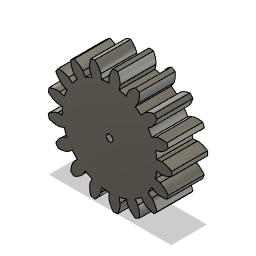
Gear v1 (Autodesk Fusion 360 design; units mm, degrees)
Autodesk Fusion 360 part; units mm, degrees
note: some values were not read from the file. Set by a fixed rule: which sketch regions a step uses.
(part 1 of 6)
sketch "Sketch1" plane through (0, 0, 0) normal (0, 0, 1) x (1, 0, 0)
  spline S0 degree 5 poles (16.3808, -1.6095) (16.3809, -1.6096) (16.3812, -1.6096) (16.3817, -1.6096) (16.3824, -1.6097) (16.3835, -1.6098) (16.3848, -1.6099) (16.3862, -1.61) (16.3879, -1.6101) (16.3897, -1.6102) (16.3916, -1.6103) (16.3937, -1.6104) (16.396, -1.6106) (16.3984, -1.6107) (16.401, -1.6108) (16.4037, -1.6109) (16.4066, -1.6111) (16.4096, -1.6112) (16.4128, -1.6113) (16.4161, -1.6114) (16.4195, -1.6115) (16.4231, -1.6116) (16.4268, -1.6117) (16.4306, -1.6118) (16.4346, -1.6118) (16.4387, -1.6119) (16.443, -1.6119) (16.4473, -1.612) (16.4518, -1.612) (16.4564, -1.612) (16.4611, -1.612) (16.466, -1.612) (16.471, -1.612) (16.476, -1.6119) (16.4812, -1.6119) (16.4866, -1.6118) (16.492, -1.6117) (16.4975, -1.6116) (16.5032, -1.6115) (16.5089, -1.6113) (16.5148, -1.6111) (16.5207, -1.6109) (16.5268, -1.6107) (16.533, -1.6105) (16.5393, -1.6103) (16.5456, -1.61) (16.5521, -1.6097) (16.5587, -1.6094) (16.5654, -1.609) (16.5722, -1.6087) (16.579, -1.6083) (16.586, -1.6079) (16.5931, -1.6074) (16.6002, -1.607) (16.6075, -1.6065) (16.6148, -1.606) (16.6222, -1.6054) (16.6298, -1.6049) (16.6374, -1.6043) (16.6451, -1.6036) (16.6528, -1.603) (16.6607, -1.6023) (16.6687, -1.6016) (16.6767, -1.6009) (16.6848, -1.6001) (16.693, -1.5993) (16.7013, -1.5985) (16.7097, -1.5977) (16.7181, -1.5968) (16.7267, -1.5959) (16.7353, -1.5949) (16.744, -1.594) (16.7527, -1.593) (16.7616, -1.5919) (16.7705, -1.5909) (16.7795, -1.5898) (16.7885, -1.5886) (16.7977, -1.5875) (16.8069, -1.5863) (16.8162, -1.585) (16.8256, -1.5838) (16.835, -1.5825) (16.8445, -1.5812) (16.8541, -1.5798) (16.8637, -1.5784) (16.8734, -1.577) (16.8832, -1.5755) (16.8931, -1.574) (16.903, -1.5725) (16.913, -1.5709) (16.923, -1.5693) (16.9331, -1.5676) (16.9433, -1.566) (16.9536, -1.5643) (16.9639, -1.5625) (16.9742, -1.5607) (16.9847, -1.5589) (16.9952, -1.557) (17.0057, -1.5552) (17.0164, -1.5532) (17.0271, -1.5512) (17.0378, -1.5492) (17.0486, -1.5472) (17.0595, -1.5451) (17.0704, -1.543) (17.0814, -1.5408) (17.0924, -1.5386) (17.1035, -1.5364) (17.1147, -1.5341) (17.1259, -1.5318) (17.1372, -1.5295) (17.1485, -1.5271) (17.1599, -1.5247) (17.1713, -1.5222) (17.1828, -1.5197) (17.1944, -1.5171) (17.206, -1.5146) (17.2176, -1.5119) (17.2293, -1.5093) (17.2411, -1.5066) (17.2529, -1.5038) (17.2647, -1.501) (17.2767, -1.4982) (17.2886, -1.4953) (17.3006, -1.4924) (17.3127, -1.4895) (17.3248, -1.4865) (17.337, -1.4835) (17.3492, -1.4804) (17.3614, -1.4773) (17.3738, -1.4741) (17.3861, -1.4709) (17.3985, -1.4677) (17.411, -1.4644) (17.4235, -1.4611) (17.436, -1.4578) (17.4486, -1.4544) (17.4612, -1.4509) (17.4739, -1.4474) (17.4866, -1.4439) (17.4994, -1.4403) (17.5122, -1.4367) (17.5251, -1.4331) (17.538, -1.4294) (17.5509, -1.4256) (17.5639, -1.4218) (17.5769, -1.418) (17.59, -1.4141) (17.6031, -1.4102) (17.6163, -1.4063) (17.6295, -1.4023) (17.6427, -1.3982) (17.656, -1.3942) (17.6693, -1.39) (17.6827, -1.3859) (17.696, -1.3816) (17.7095, -1.3774) (17.723, -1.3731) (17.7365, -1.3687) (17.75, -1.3643) (17.7636, -1.3599) (17.7772, -1.3554) (17.7909, -1.3509) (17.8046, -1.3463) (17.8183, -1.3417) (17.8321, -1.3371) (17.8459, -1.3324) (17.8598, -1.3276) (17.8736, -1.3229) (17.8876, -1.318) (17.9015, -1.3131) (17.9155, -1.3082) (17.9295, -1.3033) (17.9436, -1.2982) (17.9577, -1.2932) (17.9718, -1.2881) (17.9859, -1.283) (18.0001, -1.2778) (18.0143, -1.2725) (18.0286, -1.2672) (18.0429, -1.2619) (18.0572, -1.2566) (18.0716, -1.2511) (18.0859, -1.2457) (18.1004, -1.2402) (18.1148, -1.2346) (18.1293, -1.229) (18.1438, -1.2234) (18.1583, -1.2177) (18.1729, -1.212) (18.1875, -1.2062) (18.2021, -1.2004) (18.2167, -1.1945) (18.2314, -1.1886) (18.2461, -1.1826) (18.2609, -1.1766) (18.2756, -1.1706) (18.2904, -1.1645) (18.3053, -1.1583) (18.3201, -1.1521) (18.335, -1.1459) (18.3499, -1.1396) (18.3648, -1.1333) (18.3798, -1.1269) (18.3948, -1.1205) (18.4098, -1.114) (18.4248, -1.1075) (18.4399, -1.101) (18.4549, -1.0943) (18.4701, -1.0877) (18.4852, -1.081) (18.5004, -1.0743) (18.5155, -1.0675) (18.5307, -1.0606) (18.546, -1.0537) (18.5612, -1.0468) (18.5765, -1.0398) (18.5918, -1.0328) (18.6071, -1.0257) (18.6225, -1.0186) (18.6379, -1.0115) (18.6533, -1.0043) (18.6687, -0.997) (18.6841, -0.9897) (18.6996, -0.9824) (18.7151, -0.975) (18.7306, -0.9675) (18.7461, -0.96) (18.7616, -0.9525) (18.7772, -0.9449) (18.7928, -0.9373) (18.8084, -0.9296) (18.824, -0.9219) (18.8397, -0.9141) (18.8553, -0.9063) (18.871, -0.8984) (18.8867, -0.8905) (18.9024, -0.8826) (18.9182, -0.8746) (18.9339, -0.8665) (18.9497, -0.8584) (18.9624, -0.8519) (18.9718, -0.847) (18.9782, -0.8437) (18.9813, -0.8421) knots 0 0 0 0 0 0 0.00416667 0.00833333 0.0125 0.01666667 0.02083333 0.025 0.02916667 0.03333333 0.0375 0.04166667 0.04583333 0.05 0.05416667 0.05833333 0.0625 0.06666667 0.07083333 0.075 0.07916667 0.08333333 0.0875 0.09166667 0.09583333 0.1 0.10416667 0.10833333 0.1125 0.11666667 0.12083333 0.125 0.12916667 0.13333333 0.1375 0.14166667 0.14583333 0.15 0.15416667 0.15833333 0.1625 0.16666667 0.17083333 0.175 0.17916667 0.18333333 0.1875 0.19166667 0.19583333 0.2 0.20416667 0.20833333 0.2125 0.21666667 0.22083333 0.225 0.22916667 0.23333333 0.2375 0.24166667 0.24583333 0.25 0.25416667 0.25833333 0.2625 0.26666667 0.27083333 0.275 0.27916667 0.28333333 0.2875 0.29166667 0.29583333 0.3 0.30416667 0.30833333 0.3125 0.31666667 0.32083333 0.325 0.32916667 0.33333333 0.3375 0.34166667 0.34583333 0.35 0.35416667 0.35833333 0.3625 0.36666667 0.37083333 0.375 0.37916667 0.38333333 0.3875 0.39166667 0.39583333 0.4 0.40416667 0.40833333 0.4125 0.41666667 0.42083333 0.425 0.42916667 0.43333333 0.4375 0.44166667 0.44583333 0.45 0.45416667 0.45833333 0.4625 0.46666667 0.47083333 0.475 0.47916667 0.48333333 0.4875 0.49166667 0.49583333 0.5 0.50416667 0.50833333 0.5125 0.51666667 0.52083333 0.525 0.52916667 0.53333333 0.5375 0.54166667 0.54583333 0.55 0.55416667 0.55833333 0.5625 0.56666667 0.57083333 0.575 0.57916667 0.58333333 0.5875 0.59166667 0.59583333 0.6 0.60416667 0.60833333 0.6125 0.61666667 0.62083333 0.625 0.62916667 0.63333333 0.6375 0.64166667 0.64583333 0.65 0.65416667 0.65833333 0.6625 0.66666667 0.67083333 0.675 0.67916667 0.68333333 0.6875 0.69166667 0.69583333 0.7 0.70416667 0.70833333 0.7125 0.71666667 0.72083333 0.725 0.72916667 0.73333333 0.7375 0.74166667 0.74583333 0.75 0.75416667 0.75833333 0.7625 0.76666667 0.77083333 0.775 0.77916667 0.78333333 0.7875 0.79166667 0.79583333 0.8 0.80416667 0.80833333 0.8125 0.81666667 0.82083333 0.825 0.82916667 0.83333333 0.8375 0.84166667 0.84583333 0.85 0.85416667 0.85833333 0.8625 0.86666667 0.87083333 0.875 0.87916667 0.88333333 0.8875 0.89166667 0.89583333 0.9 0.90416667 0.90833333 0.9125 0.91666667 0.92083333 0.925 0.92916667 0.93333333 0.9375 0.94166667 0.94583333 0.95 0.95416667 0.95833333 0.9625 0.96666667 0.97083333 0.975 0.97916667 0.98333333 0.9875 0.99166667 0.99583333 1 1 1 1 1 1
  spline S1 degree 5 poles (16.3808, 1.6095) (16.3809, 1.6096) (16.3812, 1.6096) (16.3817, 1.6096) (16.3824, 1.6097) (16.3835, 1.6098) (16.3848, 1.6099) (16.3862, 1.61) (16.3879, 1.6101) (16.3897, 1.6102) (16.3916, 1.6103) (16.3937, 1.6104) (16.396, 1.6106) (16.3984, 1.6107) (16.401, 1.6108) (16.4037, 1.6109) (16.4066, 1.6111) (16.4096, 1.6112) (16.4128, 1.6113) (16.4161, 1.6114) (16.4195, 1.6115) (16.4231, 1.6116) (16.4268, 1.6117) (16.4306, 1.6118) (16.4346, 1.6118) (16.4387, 1.6119) (16.443, 1.6119) (16.4473, 1.612) (16.4518, 1.612) (16.4564, 1.612) (16.4611, 1.612) (16.466, 1.612) (16.471, 1.612) (16.476, 1.6119) (16.4812, 1.6119) (16.4866, 1.6118) (16.492, 1.6117) (16.4975, 1.6116) (16.5032, 1.6115) (16.5089, 1.6113) (16.5148, 1.6111) (16.5207, 1.6109) (16.5268, 1.6107) (16.533, 1.6105) (16.5393, 1.6103) (16.5456, 1.61) (16.5521, 1.6097) (16.5587, 1.6094) (16.5654, 1.609) (16.5722, 1.6087) (16.579, 1.6083) (16.586, 1.6079) (16.5931, 1.6074) (16.6002, 1.607) (16.6075, 1.6065) (16.6148, 1.606) (16.6222, 1.6054) (16.6298, 1.6049) (16.6374, 1.6043) (16.6451, 1.6036) (16.6528, 1.603) (16.6607, 1.6023) (16.6687, 1.6016) (16.6767, 1.6009) (16.6848, 1.6001) (16.693, 1.5993) (16.7013, 1.5985) (16.7097, 1.5977) (16.7181, 1.5968) (16.7267, 1.5959) (16.7353, 1.5949) (16.744, 1.594) (16.7527, 1.593) (16.7616, 1.5919) (16.7705, 1.5909) (16.7795, 1.5898) (16.7885, 1.5886) (16.7977, 1.5875) (16.8069, 1.5863) (16.8162, 1.585) (16.8256, 1.5838) (16.835, 1.5825) (16.8445, 1.5812) (16.8541, 1.5798) (16.8637, 1.5784) (16.8734, 1.577) (16.8832, 1.5755) (16.8931, 1.574) (16.903, 1.5725) (16.913, 1.5709) (16.923, 1.5693) (16.9331, 1.5676) (16.9433, 1.566) (16.9536, 1.5643) (16.9639, 1.5625) (16.9742, 1.5607) (16.9847, 1.5589) (16.9952, 1.557) (17.0057, 1.5552) (17.0164, 1.5532) (17.0271, 1.5512) (17.0378, 1.5492) (17.0486, 1.5472) (17.0595, 1.5451) (17.0704, 1.543) (17.0814, 1.5408) (17.0924, 1.5386) (17.1035, 1.5364) (17.1147, 1.5341) (17.1259, 1.5318) (17.1372, 1.5295) (17.1485, 1.5271) (17.1599, 1.5247) (17.1713, 1.5222) (17.1828, 1.5197) (17.1944, 1.5171) (17.206, 1.5146) (17.2176, 1.5119) (17.2293, 1.5093) (17.2411, 1.5066) (17.2529, 1.5038) (17.2647, 1.501) (17.2767, 1.4982) (17.2886, 1.4953) (17.3006, 1.4924) (17.3127, 1.4895) (17.3248, 1.4865) (17.337, 1.4835) (17.3492, 1.4804) (17.3614, 1.4773) (17.3738, 1.4741) (17.3861, 1.4709) (17.3985, 1.4677) (17.411, 1.4644) (17.4235, 1.4611) (17.436, 1.4578) (17.4486, 1.4544) (17.4612, 1.4509) (17.4739, 1.4474) (17.4866, 1.4439) (17.4994, 1.4403) (17.5122, 1.4367) (17.5251, 1.4331) (17.538, 1.4294) (17.5509, 1.4256) (17.5639, 1.4218) (17.5769, 1.418) (17.59, 1.4141) (17.6031, 1.4102) (17.6163, 1.4063) (17.6295, 1.4023) (17.6427, 1.3982) (17.656, 1.3942) (17.6693, 1.39) (17.6827, 1.3859) (17.696, 1.3816) (17.7095, 1.3774) (17.723, 1.3731) (17.7365, 1.3687) (17.75, 1.3643) (17.7636, 1.3599) (17.7772, 1.3554) (17.7909, 1.3509) (17.8046, 1.3463) (17.8183, 1.3417) (17.8321, 1.3371) (17.8459, 1.3324) (17.8598, 1.3276) (17.8736, 1.3229) (17.8876, 1.318) (17.9015, 1.3131) (17.9155, 1.3082) (17.9295, 1.3033) (17.9436, 1.2982) (17.9577, 1.2932) (17.9718, 1.2881) (17.9859, 1.283) (18.0001, 1.2778) (18.0143, 1.2725) (18.0286, 1.2672) (18.0429, 1.2619) (18.0572, 1.2566) (18.0716, 1.2511) (18.0859, 1.2457) (18.1004, 1.2402) (18.1148, 1.2346) (18.1293, 1.229) (18.1438, 1.2234) (18.1583, 1.2177) (18.1729, 1.212) (18.1875, 1.2062) (18.2021, 1.2004) (18.2167, 1.1945) (18.2314, 1.1886) (18.2461, 1.1826) (18.2609, 1.1766) (18.2756, 1.1706) (18.2904, 1.1645) (18.3053, 1.1583) (18.3201, 1.1521) (18.335, 1.1459) (18.3499, 1.1396) (18.3648, 1.1333) (18.3798, 1.1269) (18.3948, 1.1205) (18.4098, 1.114) (18.4248, 1.1075) (18.4399, 1.101) (18.4549, 1.0943) (18.4701, 1.0877) (18.4852, 1.081) (18.5004, 1.0743) (18.5155, 1.0675) (18.5307, 1.0606) (18.546, 1.0537) (18.5612, 1.0468) (18.5765, 1.0398) (18.5918, 1.0328) (18.6071, 1.0257) (18.6225, 1.0186) (18.6379, 1.0115) (18.6533, 1.0043) (18.6687, 0.997) (18.6841, 0.9897) (18.6996, 0.9824) (18.7151, 0.975) (18.7306, 0.9675) (18.7461, 0.96) (18.7616, 0.9525) (18.7772, 0.9449) (18.7928, 0.9373) (18.8084, 0.9296) (18.824, 0.9219) (18.8397, 0.9141) (18.8553, 0.9063) (18.871, 0.8984) (18.8867, 0.8905) (18.9024, 0.8826) (18.9182, 0.8746) (18.9339, 0.8665) (18.9497, 0.8584) (18.9624, 0.8519) (18.9718, 0.847) (18.9782, 0.8437) (18.9813, 0.8421) knots 0 0 0 0 0 0 0.00416667 0.00833333 0.0125 0.01666667 0.02083333 0.025 0.02916667 0.03333333 0.0375 0.04166667 0.04583333 0.05 0.05416667 0.05833333 0.0625 0.06666667 0.07083333 0.075 0.07916667 0.08333333 0.0875 0.09166667 0.09583333 0.1 0.10416667 0.10833333 0.1125 0.11666667 0.12083333 0.125 0.12916667 0.13333333 0.1375 0.14166667 0.14583333 0.15 0.15416667 0.15833333 0.1625 0.16666667 0.17083333 0.175 0.17916667 0.18333333 0.1875 0.19166667 0.19583333 0.2 0.20416667 0.20833333 0.2125 0.21666667 0.22083333 0.225 0.22916667 0.23333333 0.2375 0.24166667 0.24583333 0.25 0.25416667 0.25833333 0.2625 0.26666667 0.27083333 0.275 0.27916667 0.28333333 0.2875 0.29166667 0.29583333 0.3 0.30416667 0.30833333 0.3125 0.31666667 0.32083333 0.325 0.32916667 0.33333333 0.3375 0.34166667 0.34583333 0.35 0.35416667 0.35833333 0.3625 0.36666667 0.37083333 0.375 0.37916667 0.38333333 0.3875 0.39166667 0.39583333 0.4 0.40416667 0.40833333 0.4125 0.41666667 0.42083333 0.425 0.42916667 0.43333333 0.4375 0.44166667 0.44583333 0.45 0.45416667 0.45833333 0.4625 0.46666667 0.47083333 0.475 0.47916667 0.48333333 0.4875 0.49166667 0.49583333 0.5 0.50416667 0.50833333 0.5125 0.51666667 0.52083333 0.525 0.52916667 0.53333333 0.5375 0.54166667 0.54583333 0.55 0.55416667 0.55833333 0.5625 0.56666667 0.57083333 0.575 0.57916667 0.58333333 0.5875 0.59166667 0.59583333 0.6 0.60416667 0.60833333 0.6125 0.61666667 0.62083333 0.625 0.62916667 0.63333333 0.6375 0.64166667 0.64583333 0.65 0.65416667 0.65833333 0.6625 0.66666667 0.67083333 0.675 0.67916667 0.68333333 0.6875 0.69166667 0.69583333 0.7 0.70416667 0.70833333 0.7125 0.71666667 0.72083333 0.725 0.72916667 0.73333333 0.7375 0.74166667 0.74583333 0.75 0.75416667 0.75833333 0.7625 0.76666667 0.77083333 0.775 0.77916667 0.78333333 0.7875 0.79166667 0.79583333 0.8 0.80416667 0.80833333 0.8125 0.81666667 0.82083333 0.825 0.82916667 0.83333333 0.8375 0.84166667 0.84583333 0.85 0.85416667 0.85833333 0.8625 0.86666667 0.87083333 0.875 0.87916667 0.88333333 0.8875 0.89166667 0.89583333 0.9 0.90416667 0.90833333 0.9125 0.91666667 0.92083333 0.925 0.92916667 0.93333333 0.9375 0.94166667 0.94583333 0.95 0.95416667 0.95833333 0.9625 0.96666667 0.97083333 0.975 0.97916667 0.98333333 0.9875 0.99166667 0.99583333 1 1 1 1 1 1
  spline S2 degree 5 poles (16.3796, -1.6094) (16.3797, -1.6095) (16.3798, -1.6095) (16.3799, -1.6095) (16.3801, -1.6095) (16.3803, -1.6095) (16.3805, -1.6095) (16.3806, -1.6095) (16.3807, -1.6095) (16.3808, -1.6095) knots 0 0 0 0 0 0 0.2 0.4 0.6 0.8 1 1 1 1 1 1
  spline S3 degree 5 poles (16.3796, 1.6094) (16.3797, 1.6095) (16.3798, 1.6095) (16.3799, 1.6095) (16.3801, 1.6095) (16.3803, 1.6095) (16.3805, 1.6095) (16.3806, 1.6095) (16.3807, 1.6095) (16.3808, 1.6095) knots 0 0 0 0 0 0 0.2 0.4 0.6 0.8 1 1 1 1 1 1
  line L0 (0, 0) -> (16.3796, -1.6094)
  line L1 (0, 0) -> (16.3796, 1.6094)
  arc A0 (18.9813, -0.8421) -> (18.9813, 0.8421) centre (0, 0) ccw
  point P0 (16.3842, -1.6098)
  point P1 (16.3899, -1.6102)
  point P2 (16.3978, -1.6107)
  point P3 (16.4081, -1.6111)
  point P4 (16.4206, -1.6115)
  point P5 (16.4354, -1.6118)
  point P6 (16.4525, -1.612)
  point P7 (16.4719, -1.612)
  point P8 (16.4936, -1.6117)
  point P9 (16.5175, -1.611)
  point P10 (16.5437, -1.6101)
  point P11 (16.5722, -1.6087)
  point P12 (16.6029, -1.6068)
  point P13 (16.6359, -1.6044)
  point P14 (16.6711, -1.6014)
  point P15 (16.7086, -1.5978)
  point P16 (16.7483, -1.5935)
  point P17 (16.7901, -1.5884)
  point P18 (16.8342, -1.5826)
  point P19 (16.8805, -1.5759)
  point P20 (16.9289, -1.5683)
  point P21 (16.9795, -1.5598)
  point P22 (17.0323, -1.5503)
  point P23 (17.0871, -1.5397)
  point P24 (17.1441, -1.528)
  point P25 (17.2032, -1.5152)
  point P26 (17.2643, -1.5011)
  point P27 (17.3274, -1.4858)
  point P28 (17.3926, -1.4692)
  point P29 (17.4598, -1.4513)
  point P30 (17.529, -1.4319)
  point P31 (17.6001, -1.4111)
  point P32 (17.6732, -1.3888)
  point P33 (17.7482, -1.3649)
  point P34 (17.825, -1.3395)
  point P35 (17.9037, -1.3124)
  point P36 (17.9842, -1.2836)
  point P37 (18.0666, -1.253)
  point P38 (18.1506, -1.2207)
  point P39 (18.2365, -1.1865)
  point P40 (18.324, -1.1505)
  point P41 (18.4131, -1.1126)
  point P42 (18.504, -1.0726)
  point P43 (18.5964, -1.0307)
  point P44 (18.6904, -0.9867)
  point P45 (18.7859, -0.9407)
  point P46 (18.8829, -0.8925)
  point P47 (16.3842, 1.6098)
  point P48 (16.3899, 1.6102)
  point P49 (16.3978, 1.6107)
  point P50 (16.4081, 1.6111)
  point P51 (16.4206, 1.6115)
  point P52 (16.4354, 1.6118)
  point P53 (16.4525, 1.612)
  point P54 (16.4719, 1.612)
  point P55 (16.4936, 1.6117)
  point P56 (16.5175, 1.611)
  point P57 (16.5437, 1.6101)
  point P58 (16.5722, 1.6087)
  point P59 (16.6029, 1.6068)
  point P60 (16.6359, 1.6044)
  point P61 (16.6711, 1.6014)
  point P62 (16.7086, 1.5978)
  point P63 (16.7483, 1.5935)
  point P64 (16.7901, 1.5884)
  point P65 (16.8342, 1.5826)
  point P66 (16.8805, 1.5759)
  point P67 (16.9289, 1.5683)
  point P68 (16.9795, 1.5598)
  point P69 (17.0323, 1.5503)
  point P70 (17.0871, 1.5397)
  point P71 (17.1441, 1.528)
  point P72 (17.2032, 1.5152)
  point P73 (17.2643, 1.5011)
  point P74 (17.3274, 1.4858)
  point P75 (17.3926, 1.4692)
  point P76 (17.4598, 1.4513)
  point P77 (17.529, 1.4319)
  point P78 (17.6001, 1.4111)
  point P79 (17.6732, 1.3888)
  point P80 (17.7482, 1.3649)
  point P81 (17.825, 1.3395)
  point P82 (17.9037, 1.3124)
  point P83 (17.9842, 1.2836)
  point P84 (18.0666, 1.253)
  point P85 (18.1506, 1.2207)
  point P86 (18.2365, 1.1865)
  point P87 (18.324, 1.1505)
  point P88 (18.4131, 1.1126)
  point P89 (18.504, 1.0726)
  point P90 (18.5964, 1.0307)
  point P91 (18.6904, 0.9867)
  point P92 (18.7859, 0.9407)
  point P93 (18.8829, 0.8925)
sketch "Sketch2" plane through (0, 0, 0) normal (0, 0, 1) x (1, 0, 0)
  circle A0 centre (0, 0) radius 14.5
combine "Combine1" [no effect]
sketch "Sketch3" plane through (0, 0, 0) normal (0, 0, 1) x (1, 0, 0)
  line L0 (0, 0) -> (45.813, 0) construction
  line L1 (45.813, 0) -> (45.813, 3) construction
  line L2 (45.813, 3) -> (0, 3) construction
  line L3 (0, 3) -> (0, 0) construction
  constraint perpendicular L0 L1
  constraint parallel L0 L2
  constraint parallel L1 L3
sketch "Sketch4" plane through (0, 0, 0) normal (0, 0, 1) x (1, 0, 0)
  spline S0 degree 5 poles (7.9421, -0.8555) (7.9422, -0.8555) (7.9424, -0.8555) (7.9426, -0.8555) (7.943, -0.8556) (7.9436, -0.8556) (7.9443, -0.8557) (7.945, -0.8557) (7.9458, -0.8558) (7.9468, -0.8559) (7.9478, -0.8559) (7.9489, -0.856) (7.9501, -0.8561) (7.9513, -0.8562) (7.9527, -0.8562) (7.9541, -0.8563) (7.9556, -0.8564) (7.9572, -0.8565) (7.9588, -0.8565) (7.9606, -0.8566) (7.9624, -0.8567) (7.9643, -0.8567) (7.9662, -0.8568) (7.9683, -0.8569) (7.9704, -0.8569) (7.9726, -0.8569) (7.9748, -0.857) (7.9771, -0.857) (7.9795, -0.857) (7.982, -0.8571) (7.9846, -0.8571) (7.9872, -0.8571) (7.9899, -0.8571) (7.9926, -0.8571) (7.9954, -0.857) (7.9983, -0.857) (8.0013, -0.857) (8.0043, -0.8569) (8.0074, -0.8569) (8.0105, -0.8568) (8.0137, -0.8567) (8.017, -0.8566) (8.0203, -0.8565) (8.0237, -0.8564) (8.0272, -0.8563) (8.0307, -0.8561) (8.0343, -0.856) (8.038, -0.8558) (8.0417, -0.8556) (8.0455, -0.8554) (8.0493, -0.8552) (8.0532, -0.855) (8.0571, -0.8547) (8.0611, -0.8545) (8.0652, -0.8542) (8.0693, -0.8539) (8.0735, -0.8536) (8.0777, -0.8533) (8.082, -0.8529) (8.0863, -0.8526) (8.0907, -0.8522) (8.0952, -0.8518) (8.0997, -0.8514) (8.1043, -0.851) (8.1089, -0.8505) (8.1136, -0.8501) (8.1183, -0.8496) (8.123, -0.8491) (8.1279, -0.8486) (8.1327, -0.848) (8.1377, -0.8475) (8.1427, -0.8469) (8.1477, -0.8463) (8.1528, -0.8457) (8.1579, -0.845) (8.1631, -0.8444) (8.1683, -0.8437) (8.1736, -0.843) (8.1789, -0.8422) (8.1842, -0.8415) (8.1897, -0.8407) (8.1951, -0.8399) (8.2006, -0.8391) (8.2062, -0.8383) (8.2118, -0.8374) (8.2174, -0.8365) (8.2231, -0.8356) (8.2289, -0.8347) (8.2346, -0.8338) (8.2405, -0.8328) (8.2463, -0.8318) (8.2523, -0.8308) (8.2582, -0.8297) (8.2642, -0.8287) (8.2703, -0.8276) (8.2763, -0.8264) (8.2825, -0.8253) (8.2886, -0.8241) (8.2948, -0.8229) (8.3011, -0.8217) (8.3074, -0.8205) (8.3137, -0.8192) (8.3201, -0.8179) (8.3265, -0.8166) (8.333, -0.8152) (8.3394, -0.8139) (8.346, -0.8125) (8.3525, -0.8111) (8.3591, -0.8096) (8.3658, -0.8081) (8.3725, -0.8066) (8.3792, -0.8051) (8.386, -0.8035) (8.3927, -0.8019) (8.3996, -0.8003) (8.4064, -0.7987) (8.4134, -0.797) (8.4203, -0.7953) (8.4273, -0.7936) (8.4343, -0.7919) (8.4413, -0.7901) (8.4484, -0.7883) (8.4555, -0.7864) (8.4627, -0.7846) (8.4699, -0.7827) (8.4771, -0.7808) (8.4843, -0.7788) (8.4916, -0.7768) (8.4989, -0.7748) (8.5063, -0.7728) (8.5137, -0.7707) (8.5211, -0.7686) (8.5285, -0.7665) (8.536, -0.7643) (8.5435, -0.7622) (8.5511, -0.7599) (8.5586, -0.7577) (8.5662, -0.7554) (8.5739, -0.7531) (8.5815, -0.7508) (8.5892, -0.7484) (8.597, -0.746) (8.6047, -0.7436) (8.6125, -0.7412) (8.6203, -0.7387) (8.6281, -0.7362) (8.636, -0.7336) (8.6439, -0.7311) (8.6518, -0.7284) (8.6598, -0.7258) (8.6678, -0.7231) (8.6758, -0.7204) (8.6838, -0.7177) (8.6919, -0.7149) (8.7, -0.7122) (8.7081, -0.7093) (8.7163, -0.7065) (8.7244, -0.7036) (8.7326, -0.7007) (8.7408, -0.6977) (8.7491, -0.6947) (8.7574, -0.6917) (8.7657, -0.6887) (8.774, -0.6856) (8.7823, -0.6825) (8.7907, -0.6793) (8.7991, -0.6762) (8.8075, -0.673) (8.816, -0.6697) (8.8245, -0.6665) (8.833, -0.6632) (8.8415, -0.6598) (8.85, -0.6565) (8.8586, -0.6531) (8.8672, -0.6496) (8.8758, -0.6462) (8.8844, -0.6427) (8.8931, -0.6391) (8.9017, -0.6356) (8.9104, -0.632) (8.9191, -0.6283) (8.9279, -0.6247) (8.9366, -0.621) (8.9454, -0.6172) (8.9542, -0.6135) (8.963, -0.6097) (8.9719, -0.6058) (8.9808, -0.602) (8.9896, -0.5981) (8.9985, -0.5942) (9.0075, -0.5902) (9.0164, -0.5862) (9.0254, -0.5822) (9.0343, -0.5781) (9.0433, -0.574) (9.0524, -0.5699) (9.0614, -0.5657) (9.0705, -0.5615) (9.0795, -0.5573) (9.0886, -0.553) (9.0977, -0.5487) (9.1069, -0.5444) (9.116, -0.54) (9.1252, -0.5356) (9.1343, -0.5312) (9.1435, -0.5267) (9.1527, -0.5222) (9.162, -0.5176) (9.1712, -0.5131) (9.1805, -0.5085) (9.1898, -0.5038) (9.199, -0.4991) (9.2084, -0.4944) (9.2177, -0.4897) (9.227, -0.4849) (9.2364, -0.4801) (9.2457, -0.4752) (9.2551, -0.4704) (9.2645, -0.4654) (9.2739, -0.4605) (9.2834, -0.4555) (9.2928, -0.4505) (9.3023, -0.4454) (9.3117, -0.4403) (9.3212, -0.4352) (9.3307, -0.43) (9.3402, -0.4249) (9.3497, -0.4196) (9.3593, -0.4144) (9.3688, -0.4091) (9.3784, -0.4037) (9.3879, -0.3984) (9.3975, -0.3929) (9.4071, -0.3875) (9.4167, -0.382) (9.4264, -0.3765) (9.436, -0.371) (9.4456, -0.3654) (9.4553, -0.3598) (9.465, -0.3541) (9.4746, -0.3485) (9.4824, -0.3439) (9.4882, -0.3404) (9.4921, -0.3381) (9.494, -0.337) knots 0 0 0 0 0 0 0.00416667 0.00833333 0.0125 0.01666667 0.02083333 0.025 0.02916667 0.03333333 0.0375 0.04166667 0.04583333 0.05 0.05416667 0.05833333 0.0625 0.06666667 0.07083333 0.075 0.07916667 0.08333333 0.0875 0.09166667 0.09583333 0.1 0.10416667 0.10833333 0.1125 0.11666667 0.12083333 0.125 0.12916667 0.13333333 0.1375 0.14166667 0.14583333 0.15 0.15416667 0.15833333 0.1625 0.16666667 0.17083333 0.175 0.17916667 0.18333333 0.1875 0.19166667 0.19583333 0.2 0.20416667 0.20833333 0.2125 0.21666667 0.22083333 0.225 0.22916667 0.23333333 0.2375 0.24166667 0.24583333 0.25 0.25416667 0.25833333 0.2625 0.26666667 0.27083333 0.275 0.27916667 0.28333333 0.2875 0.29166667 0.29583333 0.3 0.30416667 0.30833333 0.3125 0.31666667 0.32083333 0.325 0.32916667 0.33333333 0.3375 0.34166667 0.34583333 0.35 0.35416667 0.35833333 0.3625 0.36666667 0.37083333 0.375 0.37916667 0.38333333 0.3875 0.39166667 0.39583333 0.4 0.40416667 0.40833333 0.4125 0.41666667 0.42083333 0.425 0.42916667 0.43333333 0.4375 0.44166667 0.44583333 0.45 0.45416667 0.45833333 0.4625 0.46666667 0.47083333 0.475 0.47916667 0.48333333 0.4875 0.49166667 0.49583333 0.5 0.50416667 0.50833333 0.5125 0.51666667 0.52083333 0.525 0.52916667 0.53333333 0.5375 0.54166667 0.54583333 0.55 0.55416667 0.55833333 0.5625 0.56666667 0.57083333 0.575 0.57916667 0.58333333 0.5875 0.59166667 0.59583333 0.6 0.60416667 0.60833333 0.6125 0.61666667 0.62083333 0.625 0.62916667 0.63333333 0.6375 0.64166667 0.64583333 0.65 0.65416667 0.65833333 0.6625 0.66666667 0.67083333 0.675 0.67916667 0.68333333 0.6875 0.69166667 0.69583333 0.7 0.70416667 0.70833333 0.7125 0.71666667 0.72083333 0.725 0.72916667 0.73333333 0.7375 0.74166667 0.74583333 0.75 0.75416667 0.75833333 0.7625 0.76666667 0.77083333 0.775 0.77916667 0.78333333 0.7875 0.79166667 0.79583333 0.8 0.80416667 0.80833333 0.8125 0.81666667 0.82083333 0.825 0.82916667 0.83333333 0.8375 0.84166667 0.84583333 0.85 0.85416667 0.85833333 0.8625 0.86666667 0.87083333 0.875 0.87916667 0.88333333 0.8875 0.89166667 0.89583333 0.9 0.90416667 0.90833333 0.9125 0.91666667 0.92083333 0.925 0.92916667 0.93333333 0.9375 0.94166667 0.94583333 0.95 0.95416667 0.95833333 0.9625 0.96666667 0.97083333 0.975 0.97916667 0.98333333 0.9875 0.99166667 0.99583333 1 1 1 1 1 1
  spline S1 degree 5 poles (7.9421, 0.8555) (7.9422, 0.8555) (7.9424, 0.8555) (7.9426, 0.8555) (7.943, 0.8556) (7.9436, 0.8556) (7.9443, 0.8557) (7.945, 0.8557) (7.9458, 0.8558) (7.9468, 0.8559) (7.9478, 0.8559) (7.9489, 0.856) (7.9501, 0.8561) (7.9513, 0.8562) (7.9527, 0.8562) (7.9541, 0.8563) (7.9556, 0.8564) (7.9572, 0.8565) (7.9588, 0.8565) (7.9606, 0.8566) (7.9624, 0.8567) (7.9643, 0.8567) (7.9662, 0.8568) (7.9683, 0.8569) (7.9704, 0.8569) (7.9726, 0.8569) (7.9748, 0.857) (7.9771, 0.857) (7.9795, 0.857) (7.982, 0.8571) (7.9846, 0.8571) (7.9872, 0.8571) (7.9899, 0.8571) (7.9926, 0.8571) (7.9954, 0.857) (7.9983, 0.857) (8.0013, 0.857) (8.0043, 0.8569) (8.0074, 0.8569) (8.0105, 0.8568) (8.0137, 0.8567) (8.017, 0.8566) (8.0203, 0.8565) (8.0237, 0.8564) (8.0272, 0.8563) (8.0307, 0.8561) (8.0343, 0.856) (8.038, 0.8558) (8.0417, 0.8556) (8.0455, 0.8554) (8.0493, 0.8552) (8.0532, 0.855) (8.0571, 0.8547) (8.0611, 0.8545) (8.0652, 0.8542) (8.0693, 0.8539) (8.0735, 0.8536) (8.0777, 0.8533) (8.082, 0.8529) (8.0863, 0.8526) (8.0907, 0.8522) (8.0952, 0.8518) (8.0997, 0.8514) (8.1043, 0.851) (8.1089, 0.8505) (8.1136, 0.8501) (8.1183, 0.8496) (8.123, 0.8491) (8.1279, 0.8486) (8.1327, 0.848) (8.1377, 0.8475) (8.1427, 0.8469) (8.1477, 0.8463) (8.1528, 0.8457) (8.1579, 0.845) (8.1631, 0.8444) (8.1683, 0.8437) (8.1736, 0.843) (8.1789, 0.8422) (8.1842, 0.8415) (8.1897, 0.8407) (8.1951, 0.8399) (8.2006, 0.8391) (8.2062, 0.8383) (8.2118, 0.8374) (8.2174, 0.8365) (8.2231, 0.8356) (8.2289, 0.8347) (8.2346, 0.8338) (8.2405, 0.8328) (8.2463, 0.8318) (8.2523, 0.8308) (8.2582, 0.8297) (8.2642, 0.8287) (8.2703, 0.8276) (8.2763, 0.8264) (8.2825, 0.8253) (8.2886, 0.8241) (8.2948, 0.8229) (8.3011, 0.8217) (8.3074, 0.8205) (8.3137, 0.8192) (8.3201, 0.8179) (8.3265, 0.8166) (8.333, 0.8152) (8.3394, 0.8139) (8.346, 0.8125) (8.3525, 0.8111) (8.3591, 0.8096) (8.3658, 0.8081) (8.3725, 0.8066) (8.3792, 0.8051) (8.386, 0.8035) (8.3927, 0.8019) (8.3996, 0.8003) (8.4064, 0.7987) (8.4134, 0.797) (8.4203, 0.7953) (8.4273, 0.7936) (8.4343, 0.7919) (8.4413, 0.7901) (8.4484, 0.7883) (8.4555, 0.7864) (8.4627, 0.7846) (8.4699, 0.7827) (8.4771, 0.7808) (8.4843, 0.7788) (8.4916, 0.7768) (8.4989, 0.7748) (8.5063, 0.7728) (8.5137, 0.7707) (8.5211, 0.7686) (8.5285, 0.7665) (8.536, 0.7643) (8.5435, 0.7622) (8.5511, 0.7599) (8.5586, 0.7577) (8.5662, 0.7554) (8.5739, 0.7531) (8.5815, 0.7508) (8.5892, 0.7484) (8.597, 0.746) (8.6047, 0.7436) (8.6125, 0.7412) (8.6203, 0.7387) (8.6281, 0.7362) (8.636, 0.7336) (8.6439, 0.7311) (8.6518, 0.7284) (8.6598, 0.7258) (8.6678, 0.7231) (8.6758, 0.7204) (8.6838, 0.7177) (8.6919, 0.7149) (8.7, 0.7122) (8.7081, 0.7093) (8.7163, 0.7065) (8.7244, 0.7036) (8.7326, 0.7007) (8.7408, 0.6977) (8.7491, 0.6947) (8.7574, 0.6917) (8.7657, 0.6887) (8.774, 0.6856) (8.7823, 0.6825) (8.7907, 0.6793) (8.7991, 0.6762) (8.8075, 0.673) (8.816, 0.6697) (8.8245, 0.6665) (8.833, 0.6632) (8.8415, 0.6598) (8.85, 0.6565) (8.8586, 0.6531) (8.8672, 0.6496) (8.8758, 0.6462) (8.8844, 0.6427) (8.8931, 0.6391) (8.9017, 0.6356) (8.9104, 0.632) (8.9191, 0.6283) (8.9279, 0.6247) (8.9366, 0.621) (8.9454, 0.6172) (8.9542, 0.6135) (8.963, 0.6097) (8.9719, 0.6058) (8.9808, 0.602) (8.9896, 0.5981) (8.9985, 0.5942) (9.0075, 0.5902) (9.0164, 0.5862) (9.0254, 0.5822) (9.0343, 0.5781) (9.0433, 0.574) (9.0524, 0.5699) (9.0614, 0.5657) (9.0705, 0.5615) (9.0795, 0.5573) (9.0886, 0.553) (9.0977, 0.5487) (9.1069, 0.5444) (9.116, 0.54) (9.1252, 0.5356) (9.1343, 0.5312) (9.1435, 0.5267) (9.1527, 0.5222) (9.162, 0.5176) (9.1712, 0.5131) (9.1805, 0.5085) (9.1898, 0.5038) (9.199, 0.4991) (9.2084, 0.4944) (9.2177, 0.4897) (9.227, 0.4849) (9.2364, 0.4801) (9.2457, 0.4752) (9.2551, 0.4704) (9.2645, 0.4654) (9.2739, 0.4605) (9.2834, 0.4555) (9.2928, 0.4505) (9.3023, 0.4454) (9.3117, 0.4403) (9.3212, 0.4352) (9.3307, 0.43) (9.3402, 0.4249) (9.3497, 0.4196) (9.3593, 0.4144) (9.3688, 0.4091) (9.3784, 0.4037) (9.3879, 0.3984) (9.3975, 0.3929) (9.4071, 0.3875) (9.4167, 0.382) (9.4264, 0.3765) (9.436, 0.371) (9.4456, 0.3654) (9.4553, 0.3598) (9.465, 0.3541) (9.4746, 0.3485) (9.4824, 0.3439) (9.4882, 0.3404) (9.4921, 0.3381) (9.494, 0.337) knots 0 0 0 0 0 0 0.00416667 0.00833333 0.0125 0.01666667 0.02083333 0.025 0.02916667 0.03333333 0.0375 0.04166667 0.04583333 0.05 0.05416667 0.05833333 0.0625 0.06666667 0.07083333 0.075 0.07916667 0.08333333 0.0875 0.09166667 0.09583333 0.1 0.10416667 0.10833333 0.1125 0.11666667 0.12083333 0.125 0.12916667 0.13333333 0.1375 0.14166667 0.14583333 0.15 0.15416667 0.15833333 0.1625 0.16666667 0.17083333 0.175 0.17916667 0.18333333 0.1875 0.19166667 0.19583333 0.2 0.20416667 0.20833333 0.2125 0.21666667 0.22083333 0.225 0.22916667 0.23333333 0.2375 0.24166667 0.24583333 0.25 0.25416667 0.25833333 0.2625 0.26666667 0.27083333 0.275 0.27916667 0.28333333 0.2875 0.29166667 0.29583333 0.3 0.30416667 0.30833333 0.3125 0.31666667 0.32083333 0.325 0.32916667 0.33333333 0.3375 0.34166667 0.34583333 0.35 0.35416667 0.35833333 0.3625 0.36666667 0.37083333 0.375 0.37916667 0.38333333 0.3875 0.39166667 0.39583333 0.4 0.40416667 0.40833333 0.4125 0.41666667 0.42083333 0.425 0.42916667 0.43333333 0.4375 0.44166667 0.44583333 0.45 0.45416667 0.45833333 0.4625 0.46666667 0.47083333 0.475 0.47916667 0.48333333 0.4875 0.49166667 0.49583333 0.5 0.50416667 0.50833333 0.5125 0.51666667 0.52083333 0.525 0.52916667 0.53333333 0.5375 0.54166667 0.54583333 0.55 0.55416667 0.55833333 0.5625 0.56666667 0.57083333 0.575 0.57916667 0.58333333 0.5875 0.59166667 0.59583333 0.6 0.60416667 0.60833333 0.6125 0.61666667 0.62083333 0.625 0.62916667 0.63333333 0.6375 0.64166667 0.64583333 0.65 0.65416667 0.65833333 0.6625 0.66666667 0.67083333 0.675 0.67916667 0.68333333 0.6875 0.69166667 0.69583333 0.7 0.70416667 0.70833333 0.7125 0.71666667 0.72083333 0.725 0.72916667 0.73333333 0.7375 0.74166667 0.74583333 0.75 0.75416667 0.75833333 0.7625 0.76666667 0.77083333 0.775 0.77916667 0.78333333 0.7875 0.79166667 0.79583333 0.8 0.80416667 0.80833333 0.8125 0.81666667 0.82083333 0.825 0.82916667 0.83333333 0.8375 0.84166667 0.84583333 0.85 0.85416667 0.85833333 0.8625 0.86666667 0.87083333 0.875 0.87916667 0.88333333 0.8875 0.89166667 0.89583333 0.9 0.90416667 0.90833333 0.9125 0.91666667 0.92083333 0.925 0.92916667 0.93333333 0.9375 0.94166667 0.94583333 0.95 0.95416667 0.95833333 0.9625 0.96666667 0.97083333 0.975 0.97916667 0.98333333 0.9875 0.99166667 0.99583333 1 1 1 1 1 1
  spline S2 degree 5 poles (7.9414, -0.8554) (7.9415, -0.8554) (7.9415, -0.8554) (7.9416, -0.8555) (7.9417, -0.8555) (7.9419, -0.8555) (7.942, -0.8555) (7.9421, -0.8555) (7.9421, -0.8555) (7.9421, -0.8555) knots 0 0 0 0 0 0 0.2 0.4 0.6 0.8 1 1 1 1 1 1
  spline S3 degree 5 poles (7.9414, 0.8554) (7.9415, 0.8554) (7.9415, 0.8554) (7.9416, 0.8555) (7.9417, 0.8555) (7.9419, 0.8555) (7.942, 0.8555) (7.9421, 0.8555) (7.9421, 0.8555) (7.9421, 0.8555) knots 0 0 0 0 0 0 0.2 0.4 0.6 0.8 1 1 1 1 1 1
  line L0 (0, 0) -> (7.9414, -0.8554)
  line L1 (0, 0) -> (7.9414, 0.8554)
  arc A0 (9.494, -0.337) -> (9.494, 0.337) centre (0, 0) ccw
  point P0 (7.9442, -0.8557)
  point P1 (7.9476, -0.8559)
  point P2 (7.9525, -0.8562)
  point P3 (7.9587, -0.8565)
  point P4 (7.9662, -0.8568)
  point P5 (7.9752, -0.857)
  point P6 (7.9855, -0.8571)
  point P7 (7.9973, -0.857)
  point P8 (8.0104, -0.8568)
  point P9 (8.0248, -0.8563)
  point P10 (8.0407, -0.8557)
  point P11 (8.0579, -0.8547)
  point P12 (8.0765, -0.8534)
  point P13 (8.0964, -0.8517)
  point P14 (8.1177, -0.8496)
  point P15 (8.1403, -0.8472)
  point P16 (8.1643, -0.8442)
  point P17 (8.1895, -0.8407)
  point P18 (8.2161, -0.8367)
  point P19 (8.244, -0.8322)
  point P20 (8.2732, -0.827)
  point P21 (8.3037, -0.8212)
  point P22 (8.3355, -0.8147)
  point P23 (8.3685, -0.8075)
  point P24 (8.4028, -0.7996)
  point P25 (8.4383, -0.7908)
  point P26 (8.475, -0.7813)
  point P27 (8.5129, -0.7709)
  point P28 (8.552, -0.7597)
  point P29 (8.5923, -0.7475)
  point P30 (8.6337, -0.7344)
  point P31 (8.6762, -0.7203)
  point P32 (8.7199, -0.7052)
  point P33 (8.7647, -0.689)
  point P34 (8.8105, -0.6718)
  point P35 (8.8574, -0.6535)
  point P36 (8.9053, -0.6341)
  point P37 (8.9543, -0.6135)
  point P38 (9.0042, -0.5916)
  point P39 (9.0551, -0.5686)
  point P40 (9.1069, -0.5443)
  point P41 (9.1597, -0.5188)
  point P42 (9.2133, -0.4919)
  point P43 (9.2678, -0.4637)
  point P44 (9.3232, -0.4341)
  point P45 (9.3793, -0.4032)
  point P46 (9.4363, -0.3708)
  point P47 (7.9442, 0.8557)
  point P48 (7.9476, 0.8559)
  point P49 (7.9525, 0.8562)
  point P50 (7.9587, 0.8565)
  point P51 (7.9662, 0.8568)
  point P52 (7.9752, 0.857)
  point P53 (7.9855, 0.8571)
  point P54 (7.9973, 0.857)
  point P55 (8.0104, 0.8568)
  point P56 (8.0248, 0.8563)
  point P57 (8.0407, 0.8557)
  point P58 (8.0579, 0.8547)
  point P59 (8.0765, 0.8534)
  point P60 (8.0964, 0.8517)
  point P61 (8.1177, 0.8496)
  point P62 (8.1403, 0.8472)
  point P63 (8.1643, 0.8442)
  point P64 (8.1895, 0.8407)
  point P65 (8.2161, 0.8367)
  point P66 (8.244, 0.8322)
  point P67 (8.2732, 0.827)
  point P68 (8.3037, 0.8212)
  point P69 (8.3355, 0.8147)
  point P70 (8.3685, 0.8075)
  point P71 (8.4028, 0.7996)
  point P72 (8.4383, 0.7908)
  point P73 (8.475, 0.7813)
  point P74 (8.5129, 0.7709)
  point P75 (8.552, 0.7597)
  point P76 (8.5923, 0.7475)
  point P77 (8.6337, 0.7344)
  point P78 (8.6762, 0.7203)
  point P79 (8.7199, 0.7052)
  point P80 (8.7647, 0.689)
  point P81 (8.8105, 0.6718)
  point P82 (8.8574, 0.6535)
  point P83 (8.9053, 0.6341)
  point P84 (8.9543, 0.6135)
  point P85 (9.0042, 0.5916)
  point P86 (9.0551, 0.5686)
  point P87 (9.1069, 0.5443)
  point P88 (9.1597, 0.5188)
  point P89 (9.2133, 0.4919)
  point P90 (9.2678, 0.4637)
  point P91 (9.3232, 0.4341)
  point P92 (9.3793, 0.4032)
  point P93 (9.4363, 0.3708)
sketch "Sketch5" plane through (0, 0, 0) normal (0, 0, 1) x (1, 0, 0)
  circle A0 centre (0, 0) radius 7.25
extrude "Extrude3" add sketch "Sketch5" along normal blind 1.5 makes body 1
extrude "Extrude4" add sketch "Sketch4" along normal blind 1.5 separate body makes body 2
pattern_circular "C-Pattern2" count 17 over 360 about axis through (0, 0, 1.75) along (0, 0, 1) of "Extrude4" makes body 3 makes body 4 makes body 5 makes body 6 makes body 7 makes body 8 makes body 9 makes body 10 makes body 11 makes body 12 makes body 13 makes body 14 makes body 15 makes body 16 makes body 17 makes body 18
combine "Combine2" operation add target body 1 tool bodies 2 3 4 5 6 7 8 9 10 11 12 13 14 15 16 17 18
sketch "Sketch6" plane through (0, 0, 0) normal (0, 0, 1) x (1, 0, 0)
  line L0 (0, 0) -> (45.813, 0) construction
  line L1 (45.813, 0) -> (45.813, 3) construction
  line L2 (45.813, 3) -> (0, 3) construction
  line L3 (0, 3) -> (0, 0) construction
  constraint perpendicular L0 L1
  constraint parallel L0 L2
  constraint parallel L1 L3
extrude "Extrude5" add 1 faces at (-1.6943, -0.4725, 1.5) along direction (0, 0, 1) blind 4 on bodies 1 bodies 1